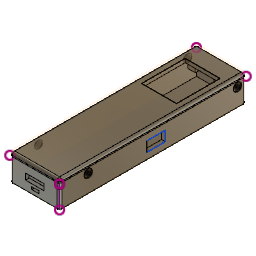
Flashlight_zhuzimo (Autodesk Fusion 360 design; units mm, degrees)
Autodesk Fusion 360 part; units mm, degrees
sketch "Sketch1" plane through (0, 0, 0) normal (0, 1, 0) x (1, 0, 0) in component "Case"
  line L0 (-20, -20) -> (20, -20)
  line L1 (20, -20) -> (20, 0)
  line L2 (20, 0) -> (-20, 0)
  line L3 (-20, 0) -> (-20, -20)
  dimension "d1" = 40
  dimension "d2" = 20
  dimension "d3" = 20
  dimension "d4" = 20
  constraint horizontal L0
  constraint vertical L1
  constraint horizontal L2
  constraint vertical L3
  measures "d1" distance of L0.start L0.end
  measures "d2" distance of L0.start L2.end
  measures "d3" vertical distance of origin L0.start
  measures "d4" horizontal distance of origin L0.start
extrude "Extrude1" add sketch "Sketch1" along normal blind 150 makes body 1 in component "Case"
fillet "Fillet1" radius 2 8 edges at (20, 0, 10) (20, 75, 0) (0, 0, 0) (-20, 0, 10) (-20, 150, 10) (0, 150, 0) (-20, 75, 0) (20, 150, 10) on bodies 1 in component "Case"
shell "Shell1" thickness 3 removed faces 1 at (-6.6667, 50.6667, 20) on bodies 1 in component "Case"
sketch "Sketch1 (2)" plane through (0, 0, 20) normal (0, 0, 1) x (-1, 0, 0) in component "Front"
  line L0 (-17, -147) -> (-17, -3)
  line L1 (-17, -3) -> (17, -3)
  line L2 (17, -3) -> (17, -147)
  line L3 (17, -147) -> (-17, -147)
  arc A0 (-18, 0) -> (-20, -2) centre (-18, -2) ccw
  line L4 (-20, -2) -> (-20, -148)
  arc A1 (-20, -148) -> (-18, -150) centre (-18, -148) ccw
  line L5 (-18, -150) -> (18, -150)
  arc A2 (18, -150) -> (20, -148) centre (18, -148) ccw
  line L6 (20, -148) -> (20, -2)
  arc A3 (20, -2) -> (18, 0) centre (18, -2) ccw
  line L7 (18, 0) -> (-18, 0)
  line L8 (17, -3) -> (-17, -3)
  line L9 (-17, -3) -> (-17, -147)
  line L10 (-17, -147) -> (17, -147)
  line L11 (17, -147) -> (17, -3)
extrude "Extrude1'" add sketch "Sketch1 (2)" along normal blind 3 separate body contours L0 L1 L2 L3 L8 L9 L10 L11 | A0 L4 A1 L5 A2 L6 A3 L7 makes body 2 in component "Front"
sketch "Sketch2" plane through (0, 0, 20) normal (0, 0, -1) x (1, 0, 0) in component "Front"
  line L0 (18, 0) -> (-18, 0)
  arc A0 (-18, 0) -> (-20, -2) centre (-18, -2) ccw
  line L1 (-20, -2) -> (-20, -148)
  arc A1 (-20, -148) -> (-18, -150) centre (-18, -148) ccw
  line L2 (-18, -150) -> (18, -150)
  arc A2 (18, -150) -> (20, -148) centre (18, -148) ccw
  line L3 (20, -148) -> (20, -2)
  arc A3 (20, -2) -> (18, 0) centre (18, -2) ccw
  line L4 (-17, -140) -> (-11, -140)
  line L5 (-11, -140) -> (-11, -146)
  line L6 (-11, -146) -> (-17, -146)
  line L7 (-17, -146) -> (-17, -140)
  line L8 (17, -140) -> (11, -140)
  line L9 (11, -140) -> (11, -146)
  line L10 (11, -146) -> (17, -146)
  line L11 (17, -146) -> (17, -140)
  line L12 (17, -20) -> (11, -20)
  line L13 (11, -20) -> (11, -26)
  line L14 (11, -26) -> (17, -26)
  line L15 (17, -26) -> (17, -20)
  line L16 (-11, -20) -> (-17, -20)
  line L17 (-17, -20) -> (-17, -26)
  line L18 (-17, -26) -> (-11, -26)
  line L19 (-11, -26) -> (-11, -20)
  dimension "d11" = 6
  dimension "d12" = 6
  dimension "d13" = 4
  dimension "d14" = 3
  dimension "d15" = 6
  dimension "d16" = 6
  dimension "d17" = 3
  dimension "d18" = 4
  dimension "d19" = 6
  dimension "d20" = 6
  dimension "d21" = 3
  dimension "d22" = 20
  dimension "d23" = 6
  dimension "d24" = 6
  dimension "d25" = 20
  dimension "d26" = 3
  constraint horizontal L4
  constraint vertical L5
  constraint horizontal L6
  constraint vertical L7
  constraint horizontal L8
  constraint vertical L9
  constraint horizontal L10
  constraint vertical L11
  constraint horizontal L12
  constraint vertical L13
  constraint horizontal L14
  constraint vertical L15
  constraint horizontal L16
  constraint vertical L17
  constraint horizontal L18
  constraint vertical L19
  measures "d11" distance of L4.start L4.end
  measures "d12" distance of L4.start L6.end
  measures "d13" vertical distance of A1.end L6.end
  measures "d14" horizontal distance of L1.end L6.end
  measures "d15" distance of L8.start L8.end
  measures "d16" distance of L8.start L10.end
  measures "d17" horizontal distance of A2.end L10.end
  measures "d18" vertical distance of L2.end L10.end
  measures "d19" distance of L12.start L12.end
  measures "d20" distance of L12.start L14.end
  measures "d21" horizontal distance of L3.end L12.start
  measures "d22" vertical distance of L0.start L12.start
  measures "d23" distance of L16.start L16.end
  measures "d24" distance of L16.start L18.end
  measures "d25" vertical distance of L0.end L16.end
  measures "d26" horizontal distance of A0.end L16.end
extrude "Extrude2" add sketch "Sketch2" along normal blind 8 contours L4 L5 L6 L7 | L8 L9 L10 L11 | L12 L13 L14 L15 | L16 L17 L18 L19 bodies 2 in component "Front"
hole "Hole1" at (-17, 143, 16) direction (1, 0, 0) diameter 2 depth 6 tip angle 118 bodies 2 in component "Front"
hole "Hole2" at (17, 143, 16) direction (-1, 0, 0) diameter 2 depth 6 tip angle 118 bodies 2 in component "Front"
hole "Hole3" at (17, 23, 16) direction (-1, 0, 0) diameter 2 depth 6 tip angle 118 bodies 2 in component "Front"
hole "Hole4" at (-17, 23, 16) direction (1, 0, 0) diameter 2 depth 6 tip angle 118 bodies 2 in component "Front"
sketch "Sketch3" plane through (0, 0, 23) normal (0, 0, 1) x (-1, 0, 0) in component "Front"
  line L0 (18, 0) -> (-18, 0)
  arc A0 (-18, 0) -> (-20, -2) centre (-18, -2) ccw
  line L1 (-20, -2) -> (-20, -148)
  arc A1 (-20, -148) -> (-18, -150) centre (-18, -148) ccw
  line L2 (-18, -150) -> (18, -150)
  arc A2 (18, -150) -> (20, -148) centre (18, -148) ccw
  line L3 (20, -148) -> (20, -2)
  arc A3 (20, -2) -> (18, 0) centre (18, -2) ccw
  line L4 (14, -135) -> (-14, -135)
  line L5 (-14, -135) -> (-14, -100)
  line L6 (-14, -100) -> (14, -100)
  line L7 (14, -100) -> (14, -135)
  dimension "d41" = 28
  dimension "d42" = 35
  dimension "d43" = 6
  dimension "d44" = 15
  constraint horizontal L4
  constraint vertical L5
  constraint horizontal L6
  constraint vertical L7
  measures "d41" distance of L4.start L4.end
  measures "d42" distance of L4.start L6.end
  measures "d43" distance of L3 L4.start
  measures "d44" vertical distance of L2.end L4.start
extrude "Extrude3" cut sketch "Sketch3" against normal blind 4 contours L4 L5 L6 L7 bodies 2 in component "Front"
sketch "Sketch2 (2)" plane through (20, 0, 0) normal (1, 0, 0) x (0, 1, 0) in component "Case"
  line L0 (2, 20) -> (2, 2)
  line L1 (2, 2) -> (148, 2)
  line L2 (148, 2) -> (148, 20)
  line L3 (148, 20) -> (2, 20)
  circle A0 centre (23, 16) radius 3.25
  circle A1 centre (143, 16) radius 3.25
  line L4 (70, 15) -> (85, 15)
  line L5 (85, 15) -> (85, 7)
  line L6 (85, 7) -> (70, 7)
  line L7 (70, 7) -> (70, 15)
  line L8 (0, 20) -> (0, 2)
  point P0 (0, 20)
  point P1 (150, 20)
  dimension "d47" = 6.5
  dimension "d48" = 4
  dimension "d49" = 23
  dimension "d50" = 6.5
  dimension "d51" = 4
  dimension "d52" = 7
  dimension "d53" = 8
  dimension "d85" = 70
  constraint horizontal L4
  constraint vertical L5
  constraint horizontal L6
  constraint vertical L7
  measures "d47" diameter of A0
  measures "d48" vertical distance of L0.start A0.centre
  measures "d49" horizontal distance of A0.centre P0
  measures "d50" diameter of A1
  measures "d51" vertical distance of L2.end A1.centre
  measures "d52" horizontal distance of A1.centre P1
  measures "d53" distance of L4.start L6.end
  measures "d85" distance of L4.start L8
hole "Hole2'" at (20, 143, 16) direction (-1, 0, 0) diameter 2 depth 6 tip angle 118 bodies 1 in component "Case"
hole "Hole1'" at (20, 23, 16) direction (-1, 0, 0) diameter 2 depth 6 tip angle 118 bodies 1 in component "Case"
extrude "Extrude2'" cut sketch "Sketch2 (2)" against normal blind 1 contours A0 | A1 bodies 1 in component "Case"
extrude "Extrude5" cut sketch "Sketch2 (2)" against normal blind 4 contours L4 L5 L6 L7 bodies 1 in component "Case"
sketch "Sketch3 (2)" plane through (-20, 0, 0) normal (-1, 0, 0) x (0, -1, 0) in component "Case"
  line L0 (-2, 2) -> (-2, 20)
  line L1 (-2, 20) -> (-148, 20)
  line L2 (-148, 20) -> (-148, 2)
  line L3 (-148, 2) -> (-2, 2)
  circle A0 centre (-143, 16) radius 3.25
  circle A1 centre (-23, 16) radius 3
  point P0 (-150, 20)
  point P1 (0, 20)
  dimension "d65" = 6.5
  dimension "d66" = 7
  dimension "d67" = 4
  dimension "d68" = 6
  dimension "d69" = 23
  dimension "d70" = 4
  measures "d65" diameter of A0
  measures "d66" horizontal distance of A0.centre P0
  measures "d67" vertical distance of L1.end A0.centre
  measures "d68" diameter of A1
  measures "d69" horizontal distance of A1.centre P1
  measures "d70" vertical distance of L0.end A1.centre
hole "Hole4'" at (-20, 143, 16) direction (1, 0, 0) diameter 2 depth 6 tip angle 118 bodies 1 in component "Case"
hole "Hole3'" at (-20, 23, 16) direction (1, 0, 0) diameter 2 depth 6 tip angle 118 bodies 1 in component "Case"
extrude "Extrude3'" cut sketch "Sketch3 (2)" against normal blind 1.5 contours A0 | A1 bodies 1 in component "Case"
sketch "Sketch4" plane through (0, 150, 0) normal (0, 1, 0) x (-1, 0, 0) in component "Case"
  line L0 (-18, 20) -> (-18, 2)
  line L1 (-18, 2) -> (18, 2)
  line L2 (18, 2) -> (18, 20)
  line L3 (18, 20) -> (-18, 20)
  circle A0 centre (0, 10) radius 4
  dimension "d79" = 8
  dimension "d80" = 10
  measures "d79" diameter of A0
  measures "d80" distance of L3 A0.centre
extrude "Extrude4" cut sketch "Sketch4" against normal blind 4 contours A0 bodies 1 in component "Case"
fillet "Fillet1'" radius 2 8 edges at (0, 150, 23) (-19.4142, 149.4142, 23) (-20, 75, 23) (-19.4142, 0.5858, 23) (0, 0, 23) (19.4142, 0.5858, 23) (20, 75, 23) (19.4142, 149.4142, 23) on bodies 2 in component "Front"
sketch "Sketch5" plane through (0, 0, 0) normal (0, -1, 0) x (1, 0, 0) in component "Case"
  line L0 (18, 2) -> (18, 20)
  line L1 (18, 20) -> (-18, 20)
  line L2 (-18, 20) -> (-18, 2)
  line L3 (-18, 2) -> (18, 2)
  line L4 (-7.5, 14) -> (7.5, 14)
  line L5 (7.5, 14) -> (7.5, 9)
  line L6 (7.5, 9) -> (-7.5, 9)
  line L7 (-7.5, 9) -> (-7.5, 14)
  line L8 (-2.5, 7) -> (3.5, 7)
  line L9 (3.5, 7) -> (3.5, 5)
  line L10 (3.5, 5) -> (-2.5, 5)
  line L11 (-2.5, 5) -> (-2.5, 7)
  line L12 (-18, 0) -> (18, 0)
  point P0 (20, 2)
  point P1 (20, 7)
  dimension "d88" = 15
  dimension "d89" = 5
  dimension "d90" = 6
  dimension "d91" = 2
  dimension "d92" = 7
  dimension "d94" = 16.5
  dimension "d95" = 9
  dimension "d96" = 12.5
  constraint horizontal L4
  constraint vertical L5
  constraint horizontal L6
  constraint vertical L7
  constraint horizontal L8
  constraint vertical L9
  constraint horizontal L10
  constraint vertical L11
  measures "d88" distance of L4.start L4.end
  measures "d89" distance of L4.start L6.end
  measures "d90" distance of L8.start L8.end
  measures "d91" distance of L8.start L10.end
  measures "d92" distance of L8.start L12
  measures "d94" distance of L8.end P1
  measures "d95" vertical distance of L5.end L12.end
  measures "d96" horizontal distance of L5.end P0
extrude "Extrude6" cut sketch "Sketch5" against normal blind 4 contours L4 L5 L6 L7 | L8 L9 L10 L11 bodies 1 in component "Case"
component "Case" placed x (1, 0, 0) y (0, 1, 0) z (0, 0, 1) at (0, 0, 0)
component "Front" placed x (1, 0, 0) y (0, 1, 0) z (0, 0, 1) at (0, 0, 0)
